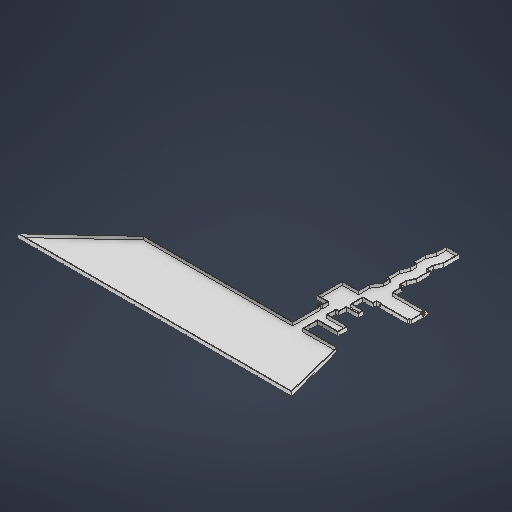
# Autodesk Inventor part: piso7
Saved by Autodesk Inventor 2026.1 (Build 301233020, 233B)
## iProperties
Created: 2025-10-08
Part Number: piso7
Material: Generic
Document SubType Name: Modeling
Designer: eduar
Density: 1 g/cm^3
Appearance: Default
Author: eduar
Autodesk Inventor part; units mm, degrees
ref_plane "YZ Plane" through (0, 0, 0) normal (1, 0, 0) x (0, 1, 0)
ref_plane "XZ Plane" through (0, 0, 0) normal (0, 1, 0) x (-1, 0, 0)
ref_plane "XY Plane" through (0, 0, 0) normal (0, 0, 1) x (1, 0, 0)
sketch "Sketch1" plane through (0, 0, 0) normal (0, 1, 0) x (-1, 0, 0)
  line L0 (0, 0) -> (0, 901.3003)
  line L1 (9787.5852, 0) -> (0, 0)
  line L2 (0, 901.3003) -> (-602.3214, 901.3003)
  line L3 (-602.3214, 901.3003) -> (-602.3214, 4403.8989)
  line L4 (0, 4403.8989) -> (-602.3214, 4403.8989)
  line L5 (0, 4403.8989) -> (0, 4821.2009)
  line L6 (8452.8733, 4821.2009) -> (0, 4821.2009)
  line L7 (8452.8733, 4821.2009) -> (8614.4121, 4641.8465)
  line L8 (9961.4788, 4641.8465) -> (8614.4121, 4641.8465)
  line L9 (9961.4788, 4641.8465) -> (9961.4788, 5800.2386)
  line L10 (9961.4788, 5800.2386) -> (13135.7444, 5800.2386)
  line L11 (13135.7444, 5800.2386) -> (13135.7444, 9607.1638)
  line L12 (13135.7444, 5800.2386) -> (9961.4788, 5800.2386)
  line L13 (13135.7444, 9607.1638) -> (13135.7444, 5800.2386)
  line L14 (13135.7444, 9607.1638) -> (9433.7487, 9607.1638)
  line L15 (9433.7487, 9607.1638) -> (9433.7487, 10999.3456)
  line L16 (13135.7444, 10999.3456) -> (9433.7487, 10999.3456)
  line L17 (13135.7444, 13359.6759) -> (13135.7444, 10999.3456)
  line L18 (13135.7444, 13359.6759) -> (14042.0345, 13359.6759)
  line L19 (14042.0345, 16368.6592) -> (14042.0345, 13359.6759)
  line L20 (7692.9526, 16368.6592) -> (14042.0345, 16368.6592)
  line L21 (7692.9526, 16368.6592) -> (7692.9526, 19092.4722)
  line L22 (14042.0345, 19092.4722) -> (7692.9526, 19092.4722)
  line L23 (14042.0345, 19092.4722) -> (14042.0345, 23788.9391)
  line L24 (14042.0345, 23788.9391) -> (3482.2606, 23788.9391)
  line L25 (-1225.0056, 42653.6139) -> (3482.2606, 23788.9391)
  line L26 (84300.724, 42653.6139) -> (-1225.0056, 42653.6139)
  line L27 (64081.9847, 23788.9391) -> (84300.724, 42653.6139)
  line L28 (17230.0732, 23788.9391) -> (64081.9847, 23788.9391)
  line L29 (17230.0732, 14918.8192) -> (17230.0732, 23788.9391)
  line L30 (18157.6351, 14918.8192) -> (17230.0732, 14918.8192)
  line L31 (18157.6351, 14490.9601) -> (18157.6351, 14918.8192)
  line L32 (17230.0732, 14490.9601) -> (18157.6351, 14490.9601)
  line L33 (17230.0732, 12465.8506) -> (17230.0732, 14490.9601)
  line L34 (20523.322, 12465.8506) -> (17230.0732, 12465.8506)
  line L35 (20523.322, 4916.0639) -> (20523.322, 12465.8506)
  line L36 (15398.5473, 4916.0639) -> (20523.322, 4916.0639)
  line L37 (15398.5473, 1338.9204) -> (15398.5473, 4916.0639)
  line L38 (15398.5473, 1338.9204) -> (13735.0003, -1130.0907)
  line L39 (13735.0003, -3413.4051) -> (13735.0003, -1130.0907)
  line L40 (14650.6953, -3413.4051) -> (13735.0003, -3413.4051)
  line L41 (14650.6953, -7235.1459) -> (14650.6953, -3413.4051)
  line L42 (14650.6953, -7235.1459) -> (13648.9917, -9727.9144)
  line L43 (13648.9917, -11709.2453) -> (13648.9917, -9727.9144)
  line L44 (13648.9917, -11709.2453) -> (14644.7947, -11709.2453)
  line L45 (14644.7947, -11709.2453) -> (14644.7947, -15475.5183)
  line L46 (14644.7947, -15475.5183) -> (13641.4468, -17943.9826)
  line L47 (13641.4468, -20887.1809) -> (13641.4468, -17943.9826)
  line L48 (13641.4468, -20887.1809) -> (9787.5852, -20887.1809)
  line L49 (9787.5852, -16147.4195) -> (9787.5852, -20887.1809)
  line L50 (10777.1765, -13774.1094) -> (9787.5852, -16147.4195)
  line L51 (10777.1765, -11709.2453) -> (10777.1765, -13774.1094)
  line L52 (9787.5852, -11709.2453) -> (10777.1765, -11709.2453)
  line L53 (9787.5852, -7645.9431) -> (9787.5852, -11709.2453)
  line L54 (9787.5852, -7645.9431) -> (10777.1765, -5263.1781)
  line L55 (10777.1765, -5263.1781) -> (10777.1765, -3413.4051)
  line L56 (10777.1765, -3413.4051) -> (10093.2065, -3413.4051)
  line L57 (10093.2065, -2855.3544) -> (10093.2065, -3413.4051)
  line L58 (10093.2065, -2855.3544) -> (9787.5852, -2855.3544)
  line L59 (9787.5852, -2855.3544) -> (9787.5852, 0)
  constraints: 120 end point, 44 perpendicular, 10 collinear, 1 horizontal
extrude "Extrusion1" add sketch "Sketch1" along normal blind 1000
shell "Shell1" thickness 200 outward yes removed faces 1 at (-49052.5677, 1000, 36365.389)
body "Solid1"
